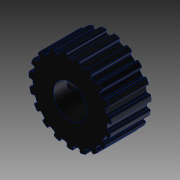
# Autodesk Inventor part: 3217b_M2Timing Belt Pulley_V1
Saved by Autodesk Inventor 2020 (Build 240168000, 168)
## iProperties
Created: 2019-11-01
Part Number: 3217b_M2Timing Belt Pulley_V1
Material: Aluminum 6061
Document SubType Name: Modeling
Designer: RFLab
Density: 2.7 g/cm^3
Appearance: Aluminum - Flat
Mass: 1.44283 g
Surface Area: 6.179 cm^2
Volume: 0.53438 cm^3
Author: RFLab
Autodesk Inventor part; units mm, degrees
ref_plane "YZ Plane" through (0, 0, 0) normal (1, 0, 0) x (0, 1, 0)
ref_plane "XZ Plane" through (0, 0, 0) normal (0, 1, 0) x (-1, 0, 0)
ref_plane "XY Plane" through (0, 0, 0) normal (0, 0, 1) x (1, 0, 0)
sketch "Sketch1" plane through (0, 0, 0) normal (0, 0, 1) x (1, 0, 0)
  circle A0 centre (0, 0) radius 6
  dimension "d0" = 12
  constraints: 1 centre point, 1 coincident
  measures "d0" diameter of A0
extrude "Extrusion1" add sketch "Sketch1" along normal mid plane 6
sketch "Sketch2" plane through (0, 0, 3) normal (0, 0, 1) x (1, 0, 0)
  circle A0 centre (0, 0) radius 6 construction
  line L0 (0, 0) -> (-0.9954, 5.9169) construction
  line L1 (-0.9954, 5.9169) -> (0.9954, 5.9169) construction
  line L2 (0.9954, 5.9169) -> (0, 0) construction
  circle A1 centre (0, 0) radius 6 construction
  line L3 (0, 5.9169) -> (0, 0) construction
  line L4 (-0.9954, 5.9169) -> (-0.4977, 5.9169)
  line L5 (-0.4977, 5.9169) -> (-0.4977, 6.2169)
  line L6 (-0.4977, 6.2169) -> (-0.9954, 6.2169) construction
  line L7 (-0.9954, 6.2169) -> (-0.9954, 5.9169) construction
  line L8 (-0.4977, 5.9169) -> (0.4977, 5.9169)
  line L9 (0.4977, 5.9169) -> (0.4977, 5.6169)
  line L10 (0.4977, 5.6169) -> (-0.4977, 5.6169)
  line L11 (-0.4977, 5.6169) -> (-0.4977, 5.9169)
  line L12 (0.4977, 5.9169) -> (0.9954, 5.9169)
  line L13 (0.9954, 5.9169) -> (0.9954, 6.2169) construction
  line L14 (0.9954, 6.2169) -> (0.4977, 6.2169) construction
  line L15 (0.4977, 6.2169) -> (0.4977, 5.9169)
  line L16 (0, 0) -> (-1.0347, 6.1503)
  circle A2 centre (0, 0) radius 6.2367
  line L17 (0, 0) -> (1.0347, 6.1503)
  point P0 (0.9954, 5.9169)
  point P1 (0.4977, 6.2169)
  point P2 (-0.9954, 5.9169)
  dimension "d4" = 0.9954
  dimension "d5" = 0.4977
  dimension "d6" = 0.3
  dimension "d7" = 0.3
  dimension "d12" = 19.099
  dimension "d13" = 9.549
  dimension "d14" = 9.549
  dimension "d15" = 1.9908
  constraints: 36 end point, 6 parallel, 5 point on circle, 3 horizontal, 3 perpendicular, 3 point on line, 1 centre point, 1 coincident, 1 midpoint, 1 vertical
  measures "d4" distance of L9.end L10.end
  measures "d5" distance of L5.end L6.end
  measures "d6" distance between parallel lines of L8 L10
  measures "d7" distance of L4.end L5.end
  measures "d12" angle of L17 L0
  measures "d13" angle of L0 L3
  measures "d14" angle of L16 L3
  measures "d15" distance of L0.end L1.end
extrude "Extrusion2" add sketch "Sketch2" against normal blind 6 contours L16 A2 L5 L4 | L15 A2 L17 L12
extrude "Extrusion3" cut sketch "Sketch2" against normal blind 6 contours L5 A2 L15 L8 | L8 L9 L10 L11
fillet "Fillet1" radius 0.2 4 edges at (-0.4977, 5.6169, 0) (-0.4977, 6.2169, 0) (0.4977, 6.2169, 0) (0.4977, 5.6169, 0)
pattern_circular "Circular Pattern1" count 19 over 360 about axis through (0, 0, 0) along (0, 0, 1) of "Extrusion3", "Extrusion2", "Fillet1"
sketch "Sketch3" plane through (0, 0, -3) normal (0, 0, -1) x (-1, 0, 0)
  circle A0 centre (0, 0) radius 2.5
  dimension "d20" = 5
  constraints: 1 centre point, 1 coincident
  measures "d20" diameter of A0
extrude "Extrusion4" cut sketch "Sketch3" against normal blind 6
sketch "Sketch4" plane through (0, 0, 0) normal (1, 0, 0) x (0, 1, 0)
  circle A0 centre (0, 0) radius 1
  dimension "d23" = 2
  constraints: 1 centre point, 1 coincident
  measures "d23" diameter of A0
extrude "Extrusion5" cut sketch "Sketch4" against normal through all
equation "\"d4\" = 0.5 * d15"
equation "\"d5\" = 0.5 * d4"
equation "\"d13\" = 0.5 * d12"
equation "\"d14\" = d13"
body "Solid1"
